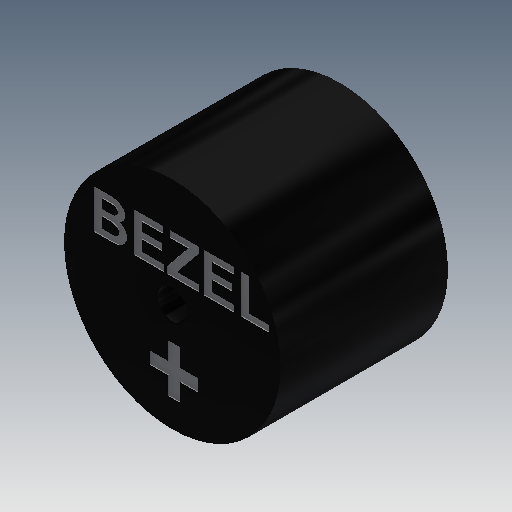
# Autodesk Inventor part: config - bezel
Saved by Autodesk Inventor 2019.1 (Build 231200000, 200)
## iProperties
Company: Autodesk Asia Pte. Ltd.
Created: 2005-12-06
Part Number: config - bezel
Document SubType Name: Modeling
Designer: Simon.Ng@autodesk.com
Stock Number: config - bezel
Density: 1 g/cm^3
Material: Generic
Mass: 0.792185 g
Surface Area: 5.23359 cm^2
Volume: 0.792185 cm^3
Appearance: Default
Title: PC Demo
Author: Simon.Ng@autodesk.com
Autodesk Inventor part; units mm, degrees
ref_plane "YZ Plane" through (0, 0, 0) normal (1, 0, 0) x (0, 1, 0)
ref_plane "XZ Plane" through (0, 0, 0) normal (0, 1, 0) x (-1, 0, 0)
ref_plane "XY Plane" through (0, 0, 0) normal (0, 0, 1) x (1, 0, 0)
sketch "Sketch1" plane through (0, 0, 0) normal (0, 0, 1) x (1, 0, 0)
  line L0 (0, 8.8) -> (0, -6.6) projected
  line L1 (-6.6, 0) -> (8.8, 0) projected
  circle A0 centre (0, 0) radius 5.5
  dimension "d0" = 11
  constraints: 2 point on line, 1 centre point
  measures "d0" diameter of A0
extrude "Extrusion1" add sketch "Sketch1" along normal blind 8.5
sketch "Sketch2" plane through (0, 0, 8.5) normal (0, 0, 1) x (1, 0, 0)
  circle A0 centre (0, 0) radius 5.5 projected
  circle A1 centre (0, 0) radius 0.75
  dimension "d3" = 1.5
  constraints: 1 centre point, 1 coincident
  measures "d3" diameter of A1
extrude "Extrusion2" cut sketch "Sketch2" against normal through all contours A1
sketch "Sketch3" plane through (0, 0, 8.5) normal (0, 0, 1) x (1, 0, 0)
  line L0 (-4.1622, 3.2044) -> (11.3317, 3.2044) construction
  line L1 (11.3317, 3.2044) -> (11.3317, -0.2956) construction
  line L2 (11.3317, -0.2956) -> (-4.1622, -0.2956) construction
  line L3 (-4.1622, -0.2956) -> (-4.1622, 3.2044) construction
  line L4 (-1.3375, -1.694) -> (1.5169, -1.694) construction
  line L5 (1.5169, -1.694) -> (1.5169, -4.135) construction
  line L6 (1.5169, -4.135) -> (-1.3375, -4.135) construction
  line L7 (-1.3375, -4.135) -> (-1.3375, -1.694) construction
  line L8 (-3.958, 3.2044) -> (-3.1577, 3.2044)
  spline S0 degree 5 poles (-3.1577, 3.2044) (-2.9199, 3.2044) (-2.6866, 3.1648) (-2.5022, 3.0398) (-2.3787, 2.8309) (-2.3787, 2.7014) knots 0 0 0 0 0 0 1 1 1 1 1 1
  spline S1 degree 3 poles (-2.3787, 2.7014) (-2.3787, 2.5611) (-2.5296, 2.3279) (-2.6592, 2.2684) knots 0 0 0 0 1 1 1 1
  spline S2 degree 3 poles (-2.6592, 2.2684) (-2.4763, 2.2151) (-2.2811, 1.959) (-2.2811, 1.7852) knots 0 0 0 0 1 1 1 1
  spline S3 degree 4 poles (-2.2811, 1.7852) (-2.2811, 1.648) (-2.4077, 1.3904) (-2.6287, 1.2364) (-2.7888, 1.2181) knots 0 0 0 0 0 1 1 1 1 1
  spline S4 degree 2 poles (-2.7888, 1.2181) (-2.8909, 1.2074) (-3.2766, 1.2044) knots 0 0 0 1 1 1
  line L9 (-3.2766, 1.2044) -> (-3.958, 1.2044)
  line L10 (-3.958, 1.2044) -> (-3.958, 3.2044)
  line L11 (-3.554, 2.0779) -> (-3.554, 1.5428)
  line L12 (-3.554, 1.5428) -> (-3.179, 1.5428)
  spline S5 degree 2 poles (-3.179, 1.5428) (-2.9595, 1.5428) (-2.9016, 1.555) knots 0 0 0 1 1 1
  spline S6 degree 3 poles (-2.9016, 1.555) (-2.8116, 1.5718) (-2.6973, 1.6983) (-2.6973, 1.805) knots 0 0 0 0 1 1 1 1
  spline S7 degree 4 poles (-2.6973, 1.805) (-2.6973, 1.8949) (-2.7842, 2.0199) (-2.9504, 2.0779) (-3.2263, 2.0779) knots 0 0 0 0 0 1 1 1 1 1
  line L13 (-3.2263, 2.0779) -> (-3.554, 2.0779)
  line L14 (-3.554, 2.8721) -> (-3.554, 2.4102)
  line L15 (-3.554, 2.4102) -> (-3.2888, 2.4102)
  spline S8 degree 2 poles (-3.2888, 2.4102) (-3.0525, 2.4102) (-2.9946, 2.4163) knots 0 0 0 1 1 1
  spline S9 degree 3 poles (-2.9946, 2.4163) (-2.8909, 2.43) (-2.772, 2.5474) (-2.772, 2.6449) knots 0 0 0 0 1 1 1 1
  spline S10 degree 3 poles (-2.772, 2.6449) (-2.772, 2.7379) (-2.8741, 2.8523) (-2.9763, 2.866) knots 0 0 0 0 1 1 1 1
  spline S11 degree 2 poles (-2.9763, 2.866) (-3.0357, 2.8721) (-3.3223, 2.8721) knots 0 0 0 1 1 1
  line L16 (-3.3223, 2.8721) -> (-3.554, 2.8721)
  line L17 (-1.9397, 1.2044) -> (-1.9397, 3.2044)
  line L18 (-1.9397, 3.2044) -> (-0.4565, 3.2044)
  line L19 (-0.4565, 3.2044) -> (-0.4565, 2.866)
  line L20 (-0.4565, 2.866) -> (-1.5357, 2.866)
  line L21 (-1.5357, 2.866) -> (-1.5357, 2.4224)
  line L22 (-1.5357, 2.4224) -> (-0.5311, 2.4224)
  line L23 (-0.5311, 2.4224) -> (-0.5311, 2.084)
  line L24 (-0.5311, 2.084) -> (-1.5357, 2.084)
  line L25 (-1.5357, 2.084) -> (-1.5357, 1.5428)
  line L26 (-1.5357, 1.5428) -> (-0.4183, 1.5428)
  line L27 (-0.4183, 1.5428) -> (-0.4183, 1.2044)
  line L28 (-0.4183, 1.2044) -> (-1.9397, 1.2044)
  line L29 (-0.2491, 1.2044) -> (-0.2491, 1.5687)
  line L30 (-0.2491, 1.5687) -> (0.8042, 2.866)
  line L31 (0.8042, 2.866) -> (-0.1302, 2.866)
  line L32 (-0.1302, 2.866) -> (-0.1302, 3.2044)
  line L33 (-0.1302, 3.2044) -> (1.3332, 3.2044)
  line L34 (1.3332, 3.2044) -> (1.3332, 2.8904)
  line L35 (1.3332, 2.8904) -> (0.2387, 1.5428)
  line L36 (0.2387, 1.5428) -> (1.3759, 1.5428)
  line L37 (1.3759, 1.5428) -> (1.3759, 1.2044)
  line L38 (1.3759, 1.2044) -> (-0.2491, 1.2044)
  line L39 (1.632, 1.2044) -> (1.632, 3.2044)
  line L40 (1.632, 3.2044) -> (3.1152, 3.2044)
  line L41 (3.1152, 3.2044) -> (3.1152, 2.866)
  line L42 (3.1152, 2.866) -> (2.0359, 2.866)
  line L43 (2.0359, 2.866) -> (2.0359, 2.4224)
  line L44 (2.0359, 2.4224) -> (3.0405, 2.4224)
  line L45 (3.0405, 2.4224) -> (3.0405, 2.084)
  line L46 (3.0405, 2.084) -> (2.0359, 2.084)
  line L47 (2.0359, 2.084) -> (2.0359, 1.5428)
  line L48 (2.0359, 1.5428) -> (3.1533, 1.5428)
  line L49 (3.1533, 1.5428) -> (3.1533, 1.2044)
  line L50 (3.1533, 1.2044) -> (1.632, 1.2044)
  line L51 (3.507, 1.2044) -> (3.507, 3.1876)
  line L52 (3.507, 3.1876) -> (3.9109, 3.1876)
  line L53 (3.9109, 3.1876) -> (3.9109, 1.5428)
  line L54 (3.9109, 1.5428) -> (4.9155, 1.5428)
  line L55 (4.9155, 1.5428) -> (4.9155, 1.2044)
  line L56 (4.9155, 1.2044) -> (3.507, 1.2044)
  line L57 (-0.2171, -4.135) -> (-0.2171, -3.2279)
  line L58 (-0.2171, -3.2279) -> (-1.1348, -3.2279)
  line L59 (-1.1348, -3.2279) -> (-1.1348, -2.601)
  line L60 (-1.1348, -2.601) -> (-0.2171, -2.601)
  line L61 (-0.2171, -2.601) -> (-0.2171, -1.694)
  line L62 (-0.2171, -1.694) -> (0.3938, -1.694)
  line L63 (0.3938, -1.694) -> (0.3938, -2.601)
  line L64 (0.3938, -2.601) -> (1.3142, -2.601)
  line L65 (1.3142, -2.601) -> (1.3142, -3.2279)
  line L66 (1.3142, -3.2279) -> (0.3938, -3.2279)
  line L67 (0.3938, -3.2279) -> (0.3938, -4.135)
  line L68 (0.3938, -4.135) -> (-0.2171, -4.135)
  constraints: 4 other
extrude "Extrusion3" cut sketch "Sketch3" against normal blind 0.05
body "Solid1"
